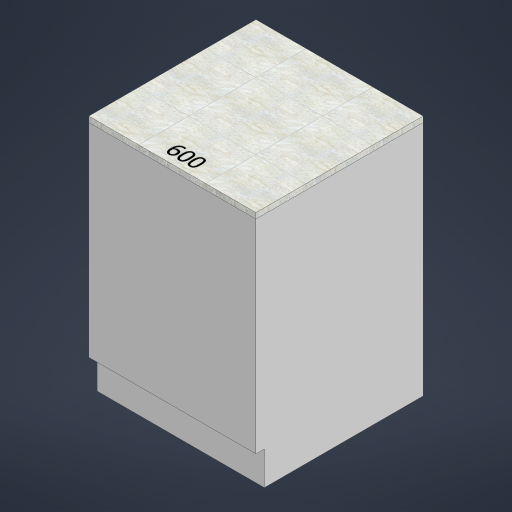
# Autodesk Inventor part: Mobile cucina
Saved by Autodesk Inventor 2025.2 (Build 292293000, 293)
## iProperties
Created: 2025-08-13
Part Number: Mobile cucina
Material: Generic
Document SubType Name: Modeling
Designer: Luca
Density: 1 g/cm^3
Appearance: Default
Mass: 311038 g
Surface Area: 35215.2 cm^2
Volume: 311038 cm^3
Author: Luca
Mass: 77758.1 g
Surface Area: 16584.3 cm^2
Volume: 77758.1 cm^3
Mass: 207358 g
Surface Area: 26935 cm^2
Volume: 207358 cm^3
Mass: 713379 g
Surface Area: 55100.2 cm^2
Volume: 713379 cm^3
Autodesk Inventor part; units mm, degrees
ref_plane "YZ Plane" through (0, 0, 0) normal (1, 0, 0) x (0, 1, 0)
ref_plane "XZ Plane" through (0, 0, 0) normal (0, 1, 0) x (-1, 0, 0)
ref_plane "XY Plane" through (0, 0, 0) normal (0, 0, 1) x (1, 0, 0)
sketch "Sketch1" plane through (0, 0, 0) normal (0, 1, 0) x (1, 0, 0)
  line L0 (300, 0) -> (-300, 0)
  line L1 (-300, 0) -> (-300, -600)
  line L2 (-300, -600) -> (300, -600)
  line L3 (300, -600) -> (300, 0)
  point P0 (0, 0)
  point P1 (0, 0)
  dimension "d0" = 600
  dimension "d1" = 600
  constraints: 8 end point, 2 parallel, 1 coincident, 1 horizontal, 1 midpoint, 1 perpendicular
  measures "d0" distance of L1.end L2.end
  measures "d1" distance of L0.end L1.end
extrude "Extrusion1" add sketch "Sketch1" along normal blind 850
sketch "Sketch2" plane through (-300, 0, 600) normal (0, 0, 1) x (-1, 0, 0)
  line L0 (-600, 0) -> (-600, -850) projected
  line L1 (0, 0) -> (0, -850) projected
  line L2 (-600, 0) -> (0, 0)
  line L3 (0, 0) -> (0, -120)
  line L4 (0, -120) -> (-600, -120)
  line L5 (-600, -120) -> (-600, 0)
  point P0 (-300, 0)
  point P1 (-600, -120)
  dimension "d4" = 120
  constraints: 8 end point, 2 parallel, 1 horizontal, 1 perpendicular, 1 point on line
  measures "d4" distance of L3.end L2.end
extrude "Extrusion2" cut sketch "Sketch2" against normal blind 30
sketch "Sketch5" plane through (0, 850, 0) normal (0, 1, 0) x (1, 0, 0)
  line L0 (300, -600) -> (300, 0) projected
  line L1 (300, 0) -> (-300, 0) projected
  line L2 (-300, 0) -> (-300, -600) projected
  line L3 (-300, -600) -> (300, -600) projected
  point P0 (0, 0)
extrude "Extrusion5" add sketch "Sketch5" along normal blind 20 separate body
sketch "Sketch6" plane through (0, 870, 0) normal (0, 1, 0) x (1, 0, 0)
  line L0 (-300, -600) -> (300, -600) projected
  line L1 (300, -600) -> (300, 0) projected
  line L2 (-300, -500) -> (300, -500) construction
  line L3 (300, -500) -> (300, -600) construction
  line L4 (300, -600) -> (-300, -600) construction
  line L5 (-300, -600) -> (-300, -500) construction
  spline S0 degree 2 poles (-21.0292, -558.7723) (-21.0292, -562.6216) (-23.5818, -569.1451) (-25.7293, -571.3331) knots 0 0 0 1 2 2 2
  spline S1 degree 2 poles (-25.7293, -571.3331) (-27.9579, -573.6426) (-33.5494, -576.0332) (-36.9125, -576.0332) knots 0 0 0 1 2 2 2
  spline S2 degree 2 poles (-36.9125, -576.0332) (-40.2755, -576.0332) (-45.8266, -573.7642) (-47.9335, -571.4951) knots 0 0 0 1 2 2 2
  spline S3 degree 2 poles (-47.9335, -571.4951) (-50.5267, -568.7804) (-53.4441, -559.6637) (-53.4441, -553.0186) knots 0 0 0 1 2 2 2
  spline S4 degree 2 poles (-53.4441, -553.0186) (-53.4441, -546.4951) (-50.7699, -536.0008) (-47.9741, -532.111) knots 0 0 0 1 2 2 2
  spline S5 degree 2 poles (-47.9741, -532.111) (-45.2593, -528.3023) (-36.6694, -524.0478) (-31.0373, -524.0478) knots 0 0 0 1 2 2 2
  spline S6 degree 2 poles (-31.0373, -524.0478) (-29.376, -524.0478) (-26.4587, -524.372) (-25.3647, -524.7366) knots 0 0 0 1 2 2 2
  line L6 (-25.3647, -524.7366) -> (-25.3647, -531.1791)
  line L7 (-25.3647, -531.1791) -> (-25.6483, -531.1791)
  spline S7 degree 2 poles (-25.6483, -531.1791) (-26.5802, -530.6929) (-29.9838, -529.842) (-31.9287, -529.842) knots 0 0 0 1 2 2 2
  spline S8 degree 2 poles (-31.9287, -529.842) (-38.1686, -529.842) (-45.8266, -538.2699) (-46.5559, -546.5357) knots 0 0 0 1 2 2 2
  spline S9 degree 2 poles (-46.5559, -546.5357) (-44.1653, -544.8744) (-39.141, -543.0511) (-36.1426, -543.0511) knots 0 0 0 1 2 2 2
  spline S10 degree 2 poles (-36.1426, -543.0511) (-33.2253, -543.0511) (-28.8493, -544.2261) (-26.4587, -546.0089) knots 0 0 0 1 2 2 2
  spline S11 degree 2 poles (-26.4587, -546.0089) (-23.7034, -548.0754) (-21.0292, -554.4773) (-21.0292, -558.7723) knots 0 0 0 1 2 2 2
  spline S12 degree 2 poles (-27.8363, -559.0559) (-27.8363, -555.9765) (-29.4571, -551.8031) (-31.2399, -550.3444) knots 0 0 0 1 2 2 2
  spline S13 degree 2 poles (-31.2399, -550.3444) (-32.577, -549.2909) (-35.8995, -548.6021) (-37.6418, -548.6021) knots 0 0 0 1 2 2 2
  spline S14 degree 2 poles (-37.6418, -548.6021) (-39.9919, -548.6021) (-44.4084, -550.0203) (-46.5559, -551.3574) knots 0 0 0 1 2 2 2
  spline S15 degree 2 poles (-46.5559, -551.3574) (-46.5964, -552.0867) (-46.6775, -553.4643) (-46.6775, -554.5178) knots 0 0 0 1 2 2 2
  spline S16 degree 2 poles (-46.6775, -554.5178) (-46.6775, -559.7042) (-44.6515, -566.0656) (-43.1118, -567.7269) knots 0 0 0 1 2 2 2
  spline S17 degree 2 poles (-43.1118, -567.7269) (-41.6937, -569.3071) (-38.6143, -570.5632) (-36.872, -570.5632) knots 0 0 0 1 2 2 2
  spline S18 degree 2 poles (-36.872, -570.5632) (-32.8201, -570.5632) (-27.8363, -564.8096) (-27.8363, -559.0559) knots 0 0 0 1 2 2 2
  spline S19 degree 2 poles (16.0049, -549.9797) (16.0049, -563.4319) (8.1848, -576.0332) (0.0405, -576.0332) knots 0 0 0 1 2 2 2
  spline S20 degree 2 poles (0.0405, -576.0332) (-8.2253, -576.0332) (-15.9643, -563.1888) (-15.9643, -550.0203) knots 0 0 0 1 2 2 2
  spline S21 degree 2 poles (-15.9643, -550.0203) (-15.9643, -536.487) (-8.1442, -523.9668) (0.0405, -523.9668) knots 0 0 0 1 2 2 2
  spline S22 degree 2 poles (0.0405, -523.9668) (8.2658, -523.9668) (16.0049, -536.9327) (16.0049, -549.9797) knots 0 0 0 1 2 2 2
  spline S23 degree 2 poles (7.4149, -565.2147) (8.3874, -562.7431) (9.1977, -555.1256) (9.1977, -549.9797) knots 0 0 0 1 2 2 2
  spline S24 degree 2 poles (9.1977, -549.9797) (9.1977, -544.8339) (8.3874, -537.2569) (7.3744, -534.7042) knots 0 0 0 1 2 2 2
  spline S25 degree 2 poles (7.3744, -534.7042) (6.3614, -532.1515) (2.8363, -529.5178) (0.0405, -529.5178) knots 0 0 0 1 2 2 2
  spline S26 degree 2 poles (0.0405, -529.5178) (-2.7553, -529.5178) (-6.3614, -532.1515) (-7.4149, -534.7853) knots 0 0 0 1 2 2 2
  spline S27 degree 2 poles (-7.4149, -534.7853) (-8.4279, -537.3379) (-9.1572, -545.1175) (-9.1572, -550.0203) knots 0 0 0 1 2 2 2
  spline S28 degree 2 poles (-9.1572, -550.0203) (-9.1572, -555.2877) (-8.5089, -562.3379) (-7.4554, -565.0932) knots 0 0 0 1 2 2 2
  spline S29 degree 2 poles (-7.4554, -565.0932) (-6.483, -567.6864) (-2.8768, -570.4822) (0.0405, -570.4822) knots 0 0 0 1 2 2 2
  spline S30 degree 2 poles (0.0405, -570.4822) (2.7958, -570.4822) (6.4019, -567.8485) (7.4149, -565.2147) knots 0 0 0 1 2 2 2
  spline S31 degree 2 poles (53.5251, -549.9797) (53.5251, -563.4319) (45.705, -576.0332) (37.5608, -576.0332) knots 0 0 0 1 2 2 2
  spline S32 degree 2 poles (37.5608, -576.0332) (29.295, -576.0332) (21.5559, -563.1888) (21.5559, -550.0203) knots 0 0 0 1 2 2 2
  spline S33 degree 2 poles (21.5559, -550.0203) (21.5559, -536.487) (29.376, -523.9668) (37.5608, -523.9668) knots 0 0 0 1 2 2 2
  spline S34 degree 2 poles (37.5608, -523.9668) (45.7861, -523.9668) (53.5251, -536.9327) (53.5251, -549.9797) knots 0 0 0 1 2 2 2
  spline S35 degree 2 poles (44.9352, -565.2147) (45.9076, -562.7431) (46.718, -555.1256) (46.718, -549.9797) knots 0 0 0 1 2 2 2
  spline S36 degree 2 poles (46.718, -549.9797) (46.718, -544.8339) (45.9076, -537.2569) (44.8947, -534.7042) knots 0 0 0 1 2 2 2
  spline S37 degree 2 poles (44.8947, -534.7042) (43.8817, -532.1515) (40.3566, -529.5178) (37.5608, -529.5178) knots 0 0 0 1 2 2 2
  spline S38 degree 2 poles (37.5608, -529.5178) (34.765, -529.5178) (31.1588, -532.1515) (30.1053, -534.7853) knots 0 0 0 1 2 2 2
  spline S39 degree 2 poles (30.1053, -534.7853) (29.0924, -537.3379) (28.363, -545.1175) (28.363, -550.0203) knots 0 0 0 1 2 2 2
  spline S40 degree 2 poles (28.363, -550.0203) (28.363, -555.2877) (29.0113, -562.3379) (30.0648, -565.0932) knots 0 0 0 1 2 2 2
  spline S41 degree 2 poles (30.0648, -565.0932) (31.0373, -567.6864) (34.6434, -570.4822) (37.5608, -570.4822) knots 0 0 0 1 2 2 2
  spline S42 degree 2 poles (37.5608, -570.4822) (40.316, -570.4822) (43.9222, -567.8485) (44.9352, -565.2147) knots 0 0 0 1 2 2 2
  point P0 (0, 0)
  dimension "d0" = 600
  dimension "d27" = 100
  constraints: 1 coincident, 1 collinear, 2 other
  measures "d27" distance of L4.end L2.start
emboss "Emboss1" sketch "Sketch6" operation cut depth 1 direction (0, -1, 0)
sketch "Sketch8" plane through (-300, 850, 600) normal (0, 0, 1) x (1, 0, 0)
  line L0 (597, 594) -> (597, 0)
  line L1 (597, 0) -> (3, 0)
  line L2 (3, 0) -> (3, 594)
  line L3 (597, 594) -> (597, 1049)
  line L4 (597, 1049) -> (3, 1049)
  line L5 (3, 1049) -> (3, 594)
  line L6 (600, -850) -> (0, -850) projected
  line L7 (0, -730) -> (600, -730) projected
  line L8 (600, -730) -> (600, 0) projected
  line L9 (0, 0) -> (600, 0) projected
  line L10 (0, -730) -> (0, 0) projected
  line L11 (600, -556) -> (600, -3)
  line L12 (600, -3) -> (0, -3)
  line L13 (0, -3) -> (0, -556)
  line L14 (0, -556) -> (0, 1052)
  line L15 (0, 1052) -> (600, 1052)
  line L16 (600, 1052) -> (600, -520.0903)
  point P0 (300, -850)
  point P1 (300, 0)
  point P2 (597, -556)
  point P3 (600, -98)
  point P4 (0, -98)
  point P5 (600, 0)
  point P6 (600, -3)
  dimension "d35" = 594
  dimension "d36" = 594
  dimension "d37" = 455
  dimension "d38" = 850
  constraints: 24 end point, 4 parallel, 3 collinear, 1 midpoint, 1 perpendicular, 1 vertical alignment, 5 other
  measures "d35" distance of L0.end L1.end
  measures "d36" distance of L0.start L0.end
  measures "d37" distance of L3.end L0.start
  measures "d38" distance between parallel lines of L1 L6
extrude "Extrusion7" [suppressed]
sketch "Sketch9" plane through (-300, 850, 600) normal (0, 0, 1) x (1, 0, 0)
  line L0 (0, -850) -> (0, 0) projected
  line L1 (0, -365) -> (600, -365)
  line L2 (600, -850) -> (600, 0) projected
  line L3 (0, 0) -> (600, 0) projected
  line L4 (0, -730) -> (600, -730) projected
  point P0 (300, -850)
  dimension "d41" = 365
  dimension "d42" = 365
  constraints: 2 end point, 2 point on line, 1 horizontal
  measures "d41" distance between parallel lines of L1 L3
  measures "d42" distance between parallel lines of L4 L1
split "Split1" [suppressed]
sketch "Sketch10" plane through (-450, 485, 600) normal (0, 0, 1) x (1, 0, 0)
  line L0 (0, -485) -> (0, 365) projected
  line L1 (0, 182.5) -> (598.7428, 182.5)
  line L2 (0, 365) -> (900, 365) projected
  line L3 (900, 0) -> (0, 0) projected
  point P0 (450, -485)
  dimension "d43" = 182.5
  dimension "d44" = 182.5
  constraints: 2 end point, 1 horizontal, 1 point on line
  measures "d43" distance between parallel lines of L1 L2
  measures "d44" distance between parallel lines of L3 L1
split "Split2" [suppressed]
sketch "Sketch3" plane through (-300, 850, 600) normal (0, 0, 1) x (1, 0, 0)
  line L0 (20, -545) -> (580, -545)
  line L1 (580, -545) -> (580, -1130)
  line L2 (580, -1130) -> (20, -1130)
  line L3 (20, -1130) -> (20, -545)
  line L4 (600, -850) -> (0, -850) projected
  point P0 (300, -850)
  point P1 (300, -1130)
  dimension "d7" = 560
  dimension "d8" = 585
  dimension "d9" = 870
  constraints: 8 end point, 2 parallel, 1 horizontal, 1 midpoint, 1 perpendicular, 1 vertical alignment
  measures "d7" distance of L1.end L2.end
  measures "d8" distance of L0.end L1.end
sketch "Sketch4" plane through (0, 850, 0) normal (0, 1, 0) x (1, 0, 0)
  line L0 (-250, 0) -> (250, 0)
  line L1 (250, 0) -> (250, -20)
  line L2 (250, -20) -> (-250, -20)
  line L3 (-250, -20) -> (-250, 0)
  line L4 (-300, 0) -> (-300, -600) projected
  line L5 (300, -600) -> (300, 0) projected
  line L6 (300, 0) -> (-300, 0) projected
  point P0 (0, 0)
  point P1 (0, 0)
  dimension "d12" = 45
  dimension "d15" = 500
  constraints: 8 end point, 2 midpoint, 2 parallel, 1 horizontal, 1 perpendicular
  measures "d15" distance of L0.start L0.end
sketch "Sketch7" plane through (-300, 850, 600) normal (0, 0, 1) x (1, 0, 0)
  line L0 (20, -510.808) -> (580, -510.808)
  line L1 (580, -510.808) -> (580, -231.235)
  line L2 (580, -231.235) -> (20, -231.235)
  line L3 (20, -231.235) -> (20, -510.808)
  line L4 (20, -1130) -> (20, -545) projected
  line L5 (580, -545) -> (580, -1130) projected
  line L6 (20, -545) -> (580, -545) projected
  point P0 (300, -850)
  dimension "d30" = 560
  dimension "d31" = 380
  dimension "d32" = 50
  constraints: 8 end point, 2 collinear, 2 parallel, 1 horizontal, 1 perpendicular
  measures "d30" distance between parallel lines of L1 L3
equation "\"d41\" = d42"
equation "\"d43\" = d44"
body "Solid1"
